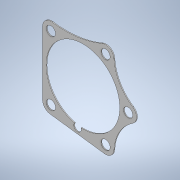
# Autodesk Inventor part: 74. Прокладка задней крышки
Saved by Autodesk Inventor 2021 (Build 250183000, 183)
## iProperties
Created: 2021-03-11
Part Number: 74. Прокладка задней крышки
Material: Типовые
Document SubType Name: Modeling
Designer: Данил
Density: 1 g/cm^3
Appearance: По умолчанию
Author: Данил
Autodesk Inventor part; units mm, degrees
ref_plane "YZ Plane" through (0, 0, 0) normal (1, 0, 0) x (0, 1, 0)
ref_plane "XZ Plane" through (0, 0, 0) normal (0, 1, 0) x (-1, 0, 0)
ref_plane "XY Plane" through (0, 0, 0) normal (0, 0, 1) x (1, 0, 0)
sketch "Эскиз1" plane through (0, 0, 0) normal (0, 0, 1) x (1, 0, 0)
  arc A0 (-2.1988, -43.945) -> (-9.9993, -42.8487) centre (0, 0) ccw
  arc A1 (-36.7231, 48.0765) -> (-48.1838, 38.1838) centre (-38.1838, 38.1838) ccw
  arc A2 (-36.7231, 48.0765) -> (23.0287, 55.943) centre (-20.6558, 156.8967) ccw
  arc A3 (36.9839, 47.3334) -> (23.0287, 55.943) centre (27, 46.7654) ccw
  arc A4 (36.9839, 47.3334) -> (59.4839, 8.3623) centre (86.9031, 50.1735) ccw
  arc A5 (59.4839, -8.3623) -> (59.4839, 8.3623) centre (54, 0) ccw
  arc A6 (59.4839, -8.3623) -> (36.9839, -47.3334) centre (86.9031, -50.1735) ccw
  arc A7 (25.6947, -56.6798) -> (36.9839, -47.3334) centre (27, -46.7654) ccw
  arc A8 (-48.1838, -38.1838) -> (-39.489, -48.0982) centre (-38.1838, -38.1838) ccw
  line L0 (-48.1838, 38.1838) -> (-48.1838, -38.1838)
  circle A9 centre (0, 0) radius 54 construction
  circle A10 centre (-38.1838, 38.1838) radius 5.5
  line L1 (0, 0) -> (-38.1838, 38.1838) construction
  line L2 (0, 0) -> (-54, 0) construction
  line L3 (0, 0) -> (27, 46.7654) construction
  line L4 (0, 0) -> (0, 54) construction
  circle A11 centre (27, 46.7654) radius 5.5
  circle A12 centre (54, 0) radius 5.5
  line L5 (0, 0) -> (-38.1838, -38.1838) construction
  line L6 (-39.489, -48.0982) -> (25.6947, -56.6798)
  line L7 (0, 0) -> (0, -54) construction
  line L8 (0, 0) -> (27, -46.7654) construction
  circle A13 centre (-38.1838, -38.1838) radius 5.5
  circle A14 centre (27, -46.7654) radius 5.5
  arc A15 (-46, 0) -> (0, -46) centre (0, 0) ccw construction
  line L9 (0, 0) -> (-6.402, -45.5523) construction
  arc A16 (-9.9993, -42.8487) -> (-2.1988, -43.945) centre (-6.402, -45.5523) ccw
  dimension "d4" = 108
  dimension "d0" = 88
  dimension "d1" = 10
  dimension "d2" = 110
  dimension "d3" = 50
  dimension "d5" = 11
  dimension "d6" = 45
  dimension "d7" = 30
  dimension "d8" = 90
  dimension "d9" = 30
  dimension "d10" = 46
  dimension "d11" = 8
  dimension "d12" = 4.5
  constraints: 23 point on circle, 20 end point, 16 centre point, 10 coincident, 10 tangent, 9 equal radius, 2 horizontal alignment, 2 vertical, 1 horizontal, 1 point on line, 1 vertical alignment, 9 other
  measures "d0" diameter of A0
  measures "d1" radius of A1
  measures "d2" radius of A2
  measures "d3" radius of A6
  measures "d5" diameter of A10
  measures "d6" angle of L2 L1
  measures "d7" angle of L4 L3
  measures "d8" angle of L5 L1
  measures "d9" angle of L7 L8
  measures "d10" radius of A15
  measures "d11" angle of L7 L9
  measures "d12" radius of A16
extrude "Выдавливание1" add sketch "Эскиз1" along normal mid plane 1
